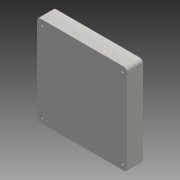
# Autodesk Inventor part: BaseFan
Saved by Autodesk Inventor 2016 (Build 200138000, 138)
## iProperties
Created: 2015-10-19
Part Number: BaseFan
Material: Generic
Document SubType Name: Modeling
Designer: Rus
Density: 1 g/cm^3
Appearance: Default
Author: Rus
Autodesk Inventor part; units mm, degrees
ref_plane "YZ Plane" through (0, 0, 0) normal (1, 0, 0) x (0, 1, 0)
ref_plane "XZ Plane" through (0, 0, 0) normal (0, 1, 0) x (-1, 0, 0)
ref_plane "XY Plane" through (0, 0, 0) normal (0, 0, 1) x (1, 0, 0)
sketch "Sketch1" plane through (0, 0, 0) normal (0, 1, 0) x (-1, 0, 0)
  line L0 (-65, 70) -> (65, 70)
  line L1 (70, 65) -> (70, -65)
  line L2 (65, -70) -> (-65, -70)
  line L3 (-70, -65) -> (-70, 65)
  line L4 (-70, 70) -> (70, -70) construction
  line L5 (70, 70) -> (-70, -70) construction
  arc A0 (70, 65) -> (65, 70) centre (65, 65) ccw
  arc A1 (-65, 70) -> (-70, 65) centre (-65, 65) ccw
  arc A2 (-70, -65) -> (-65, -70) centre (-65, -65) ccw
  arc A3 (65, -70) -> (70, -65) centre (65, -65) ccw
  line L6 (0, 70) -> (0, 62.25)
  line L7 (70, 0) -> (62.25, 0)
  line L8 (0, -70) -> (0, -62.25)
  line L9 (-70, 0) -> (-62.25, 0)
  line L10 (-62.25, 62.25) -> (-62.25, -62.25)
  line L11 (-62.25, -62.25) -> (62.25, -62.25)
  line L12 (62.25, -62.25) -> (62.25, 62.25)
  line L13 (62.25, 62.25) -> (-62.25, 62.25)
  line L14 (-62.25, 62.25) -> (62.25, -62.25) construction
  line L15 (-62.25, -62.25) -> (62.25, 62.25) construction
  circle A4 centre (62.25, -62.25) radius 2.2
  circle A5 centre (-62.25, -62.25) radius 2.2
  circle A6 centre (-62.25, 62.25) radius 2.2
  circle A7 centre (62.25, 62.25) radius 2.2
  arc A8 (60.05, 62.25) -> (62.25, 60.05) centre (62.25, 62.25) ccw
  arc A9 (62.25, -60.05) -> (60.05, -62.25) centre (62.25, -62.25) ccw
  arc A10 (-60.05, -62.25) -> (-62.25, -60.05) centre (-62.25, -62.25) ccw
  arc A11 (-62.25, 60.05) -> (-60.05, 62.25) centre (-62.25, 62.25) ccw
  arc A12 (-60.05, -62.25) -> (-62.25, -60.05) centre (-62.25, -62.25) ccw
  point P0 (0, 0)
  dimension "d0" = 140
  dimension "d1" = 140
  dimension "d2" = 5
  dimension "d3" = 7.75
  dimension "d4" = 7.75
  dimension "d5" = 7.75
  dimension "d6" = 7.75
  dimension "d7" = 4.4
  dimension "d8" = 4.4
  dimension "d9" = 4.4
  dimension "d10" = 4.4
  constraints: 32 end point, 26 point on circle, 15 point on line, 13 centre point, 10 tangent, 8 midpoint, 5 equal radius, 4 coincident, 4 parallel, 3 horizontal, 3 vertical, 2 perpendicular
  measures "d0" distance of L4.start L5.start
  measures "d1" distance of L5.start L4.end
  measures "d2" radius of A0
  measures "d3" distance of L6.start L6.end
  measures "d4" distance of L7.start L7.end
  measures "d5" distance of L8.start L8.end
  measures "d6" distance of L9.start L9.end
  measures "d7" diameter of A4
  measures "d8" diameter of A5
  measures "d9" diameter of A6
  measures "d10" diameter of A7
extrude "Extrusion1" add sketch "Sketch1" along normal blind 24.65 contours L0 L6 L13 A6 L10 L9 L3 A1 | L0 A0 L1 L7 L12 A7 L13 L6 | L13 A7 L12 A4 L11 A5 L10 A6 | L9 L10 A5 L11 L8 L2 A2 L3 | L1 A3 L2 L8 L11 A4 L12 L7 | A5 L11 L10 | L10 L11 A5
sketch "Sketch2" plane through (0, 24.65, 0) normal (0, 1, 0) x (1, 0, 0)
  circle A0 centre (62.25, -62.25) radius 2.2 projected
  line L0 (62.25, -62.25) -> (62.25, 62.25)
  line L1 (65, 70) -> (-65, 70) projected
  circle A1 centre (-62.25, 62.25) radius 2.2 projected
  line L2 (-62.25, 62.25) -> (62.25, 62.25)
  circle A2 centre (62.25, 62.25) radius 2.2
  point P0 (0, 0)
  dimension "d13" = 4.4
  constraints: 4 end point, 1 centre point, 1 coincident, 1 horizontal, 1 perpendicular
  measures "d13" diameter of A2
extrude "Extrusion2" cut sketch "Sketch2" against normal up to next contours A2 L2 L0 | L0 L2 A2
body "Solid1"
